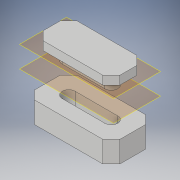
# Autodesk Inventor part: test_slot
Saved by Autodesk Inventor 2019 (Build 230136000, 136)
## iProperties
Created: 2019-05-04
Part Number: test_slot
Material: Generic
Document SubType Name: Modeling
Designer: assman
Density: 1 g/cm^3
Appearance: Default
Author: assman
## iProperties of the stored document test_slot_3DPrint.ipt
Created: 2019-05-04
Part Number: test_slot_3DPrint
Material: Generic
Document SubType Name: Modeling
Designer: assman
Density: 1 g/cm^3
Appearance: Default
Author: assman
Autodesk Inventor part; units mm, degrees
ref_plane "YZ Plane" through (0, 0, 0) normal (1, 0, 0) x (0, 1, 0)
ref_plane "XZ Plane" through (0, 0, 0) normal (0, 1, 0) x (-1, 0, 0)
ref_plane "XY Plane" through (0, 0, 0) normal (0, 0, 1) x (1, 0, 0)
sketch "Sketch1" plane through (0, 0, 0) normal (0, 1, 0) x (-1, 0, 0)
  line L0 (10, 5) -> (-10, 5)
  line L1 (-10, 5) -> (-10, -5)
  line L2 (-10, -5) -> (10, -5)
  line L3 (10, -5) -> (10, 5)
  line L4 (10, 5) -> (-10, -5) construction
  line L5 (-10, 5) -> (10, -5) construction
  point P0 (0, 0)
  dimension "d0" = 20
  dimension "d1" = 10
  constraints: 12 end point, 2 midpoint, 2 parallel, 1 horizontal, 1 perpendicular
  measures "d0" distance of L2.end L1.end
  measures "d1" distance of L1.end L0.end
extrude "Extrusion1" add sketch "Sketch1" along normal blind 5
sketch "Sketch2" plane through (0, 5, 0) normal (0, 1, 0) x (1, 0, 0)
  line L0 (-5, 0) -> (5, 0) construction
  line L1 (-5, -1.5) -> (5, -1.5)
  line L2 (5, 1.5) -> (-5, 1.5)
  arc A0 (-5, 1.5) -> (-5, -1.5) centre (-5, 0) ccw
  arc A1 (5, -1.5) -> (5, 1.5) centre (5, 0) ccw
  point P0 (0, 0)
  dimension "d4" = 5
  dimension "d5" = 3
  constraints: 8 end point, 4 point on circle, 4 tangent, 2 centre point, 1 horizontal, 1 midpoint, 1 parallel
  measures "d4" distance of point (0, 0) L0.end
  measures "d5" diameter of A1
extrude "Extrusion2" cut sketch "Sketch2" against normal blind 3
ref_plane "Work Plane1" through (0, 15, 0) normal (0, 1, 0) x (1, 0, 0)
sketch "Sketch3" plane through (0, 15, 0) normal (0, 1, 0) x (1, 0, 0)
  line L0 (-10, -5) -> (10, -5) projected
  line L1 (10, -5) -> (10, 5) projected
  line L2 (10, 5) -> (-10, 5) projected
  line L3 (-10, 5) -> (-10, -5) projected
  line L4 (5, -1.5) -> (-5, -1.5) projected
  arc A0 (5, -1.5) -> (5, 1.5) centre (5, 0) ccw projected
  line L5 (-5, 1.5) -> (5, 1.5) projected
  arc A1 (-5, 1.5) -> (-5, -1.5) centre (-5, 0) ccw projected
  point P0 (0, 0)
extrude "Extrusion3" add sketch "Sketch3" against normal blind 3 contours L4 A1 L5 A0
sketch "Sketch4" plane through (0, 15, 0) normal (0, 1, 0) x (1, 0, 0)
  line L0 (9, -4) -> (-9, -4)
  line L1 (-9, -4) -> (-9, 4)
  line L2 (-9, 4) -> (9, 4)
  line L3 (9, 4) -> (9, -4)
  line L4 (9, -4) -> (-9, 4) construction
  line L5 (-9, -4) -> (9, 4) construction
  point P0 (0, 0)
  dimension "d12" = 18
  dimension "d13" = 8
  constraints: 12 end point, 2 midpoint, 2 parallel, 1 horizontal, 1 perpendicular
  measures "d12" distance of L1.end L2.end
  measures "d13" distance of L0.end L1.end
chamfer "Chamfer1" distance 2 angle 45 4 edges at (-10, 2.5, -5) (-10, 2.5, 5) (10, 2.5, -5) (10, 2.5, 5)
extrude "Extrusion4" add sketch "Sketch4" along normal blind 2
chamfer "Chamfer2" distance 2 angle 45 4 edges at (-9, 16, -4) (-9, 16, 4) (9, 16, 4) (9, 16, -4)
ref_plane "Work Plane2" through (0, 10, 0) normal (0, 1, 0) x (1, 0, 0)
split body "Split1" result two bodies by plane through (0, 10, 0) normal (0, 1, 0) first body at (-2.3333, 16.5, 1.3333)
body "Solid2"
body "Solid3"
